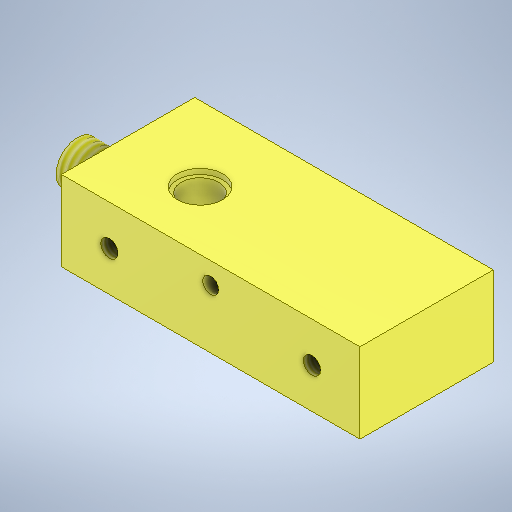
# Autodesk Inventor part: 150
Saved by Autodesk Inventor 2025.1 (Build 291241000, 241)
## iProperties
Created: 2024-08-03
Part Number: 150
Material: Steel, Cast
Document SubType Name: Modeling
Designer: ffogue
Density: 7.85 g/cm^3
Appearance: Smooth - Yellow
Author: ffogue
Autodesk Inventor part; units mm, degrees
ref_plane "YZ Plane" through (0, 0, 0) normal (1, 0, 0) x (0, 1, 0)
sketch "Sketch1" plane through (0, 0, 0) normal (0, 0, 1) x (1, 0, 0)
  line L0 (0, 0) -> (56, 0)
  line L1 (56, 0) -> (56, 25)
  line L2 (56, 25) -> (0, 25)
  line L3 (0, 25) -> (0, 0)
  dimension "d0" = 56
  dimension "d1" = 25
  constraints: 8 end point, 2 parallel, 1 horizontal, 1 perpendicular
  measures "d0" distance between parallel lines of L1 L3
  measures "d1" distance between parallel lines of L0 L2
extrude "Extrusion1" add sketch "Sketch1" along normal mid plane 15
sketch "Sketch2" plane through (0, 0, 7.5) normal (0, 0, 1) x (1, 0, 0)
  line L0 (0, 0) -> (56, 0) projected
  line L1 (0, 25) -> (0, 0) projected
  point P0 (15, 11)
  dimension "d4" = 11
  dimension "d5" = 15
  measures "d4" distance from line of L0 point (15, 11)
  measures "d5" distance from line of L1 point (15, 11)
hole "Hole1" at (15, 11, 7.5) direction (0, 0, -1) diameter 7 depth 15 counterbore diameter 8.5 counterbore depth 1
ref_plane "Work Plane1" through (0, 0, 0) normal (0, 0, 1) x (1, 0, 0)
sketch "Sketch3" plane through (0, 0, 0) normal (0, 0, 1) x (1, 0, 0)
  line L0 (1.4815, 11) -> (-8, 11)
  line L1 (-8, 11) -> (-8, 15)
  line L2 (-8, 15) -> (0, 15)
  line L3 (0, 16) -> (3, 16)
  line L4 (3, 16) -> (3, 11)
  line L5 (3, 11) -> (1.4815, 11)
  line L6 (0, 15) -> (0, 16)
  line L7 (0, 0) -> (0, 25) projected
  line L8 (56, 0) -> (0, 0) projected
  dimension "d14" = 8
  dimension "d15" = 11
  dimension "d16" = 3
  dimension "d17" = 11
  dimension "d18" = 10
  constraints: 14 end point, 4 perpendicular, 1 horizontal, 1 horizontal alignment, 1 point on line, 1 vertical, 2 other
  measures "d14" diameter of L2 L0
  measures "d15" distance between parallel lines of L4 L1
  measures "d16" distance of L3.start L3.end
  measures "d17" distance from line of L8 L4.end
  measures "d18" diameter of L3 L0
revolve "Revolution1" add sketch "Sketch3" angle 360 about axis through (1.4815, 11, 0) along (-1, 0, 0)
sketch "Sketch4" plane through (-8, 11, 0) normal (-1, 0, 0) x (0, 0, 1)
  circle A0 centre (0, 0) radius 4 projected
  point P0 (0, -11)
  constraints: 1 coincident
hole "Hole2" at (-8, 11, 0) direction (1, 0, 0) diameter 5 depth 11
thread "Thread1"
sketch "Sketch6" plane through (0, 0, 7.5) normal (0, -1, 0) x (1, 0, 0)
  line L0 (0, -15) -> (0, 0) projected
  line L1 (56, 0) -> (56, -15) projected
  line L2 (0, 0) -> (56, 0) projected
  point P0 (0, -7.5)
  point P1 (9, -7.5)
  point P2 (47, -7.5)
  point P3 (0, -7.5)
  point P4 (56, -7.5)
  point P5 (28, 0)
  dimension "d29" = 38
  dimension "d30" = 19
  constraints: 3 midpoint, 2 horizontal alignment
  measures "d29" distance of point (47, -7.5) point (9, -7.5)
  measures "d30" horizontal distance of point (28, 0) point (47, -7.5)
hole "Hole3" at (9, 0, 0) at (47, 0, 0) direction (0, 1, 0) diameter 3.242 depth 5
ref_plane "Work Plane3" through (28, 0, 7.5) normal (1, 0, 0) x (0, 0, -1)
sketch "Sketch8" plane through (28, 0, 7.5) normal (1, 0, 0) x (0, 0, -1)
  line L0 (15, 25) -> (0, 25) projected
  line L1 (15, 0) -> (15, 25) projected
  line L2 (9.8, 25) -> (4, 0)
  line L3 (0, 25) -> (0, 0) projected
  line L4 (15, 0) -> (0, 0) projected
  point P0 (7.5, 0)
  dimension "d40" = 5.2
  dimension "d41" = 4
  constraints: 2 end point, 2 point on line
  measures "d40" distance from line of L1 L2.start
  measures "d41" distance from line of L3 L2.end
sketch "Sketch10" plane through (0, 25, 7.5) normal (0, 1, 0) x (1, 0, 0)
  circle A0 centre (28, 9.8) radius 1.5
  point P0 (0, 7.5)
  dimension "d42" = 3
  constraints: 1 centre point, 1 coincident
  measures "d42" diameter of A0
sweep "Sweep1" cut profiles "Sketch10" path "Sketch8" path curves L2
sketch "Sketch12" plane through (3, 11, 0) normal (-1, 0, 0) x (0, 0, 1)
  line L0 (-7.5, 14) -> (7.5, 14) projected
  line L1 (7.5, -11) -> (7.5, 14) projected
  line L2 (7.5, -11) -> (-7.5, -11) projected
  line L3 (-7.5, 14) -> (-7.5, -11) projected
  circle A0 centre (0, 0) radius 1.5
  point P0 (0, -11)
  point P1 (0, 14)
  dimension "d45" = 3
  dimension "d46" = 11
  constraints: 1 centre point, 1 midpoint, 1 vertical alignment
  measures "d45" diameter of A0
  measures "d46" distance from line of L2 A0.centre
extrude "Extrusion2" cut sketch "Sketch12" against normal blind 32 contours A0
body "Solid1"
